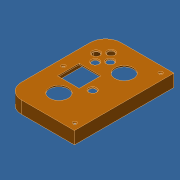
# Autodesk Inventor part: P1704_018_hautManette
Saved by Autodesk Inventor 2019 (Build 230136000, 136)
## iProperties
Created: 2019-05-28
Part Number: P1704_018_hautManette
Project: Nom Projet
Material: .
Description: Nom pièce
Document SubType Name: Modeling
Designer: Adel.KAHRIMANOVIC
Authority: brut Ø
Density: 0.001 g/cm^3
Appearance: Orange
Material number: ---
Author: Adel.KAHRIMANOVIC
Autodesk Inventor part; units mm, degrees
ref_plane "Plan YZ" through (0, 0, 0) normal (1, 0, 0) x (0, 1, 0)
ref_plane "Plan XZ" through (0, 0, 0) normal (0, 1, 0) x (-1, 0, 0)
ref_plane "Plan XY" through (0, 0, 0) normal (0, 0, 1) x (1, 0, 0)
sketch "Esquisse1" plane through (0, 0, 0) normal (0, 0, 1) x (1, 0, 0)
  line L0 (55, 80) -> (55, -80)
  line L1 (-55, -80) -> (-55, 80)
  line L2 (-55, 80) -> (55, -80) construction
  line L3 (55, 80) -> (-55, -80) construction
  line L4 (0, 0) -> (-55, 0) construction
  arc A0 (-55, -55) -> (-30, -80) centre (-30, -55) ccw
  line L5 (-30, -80) -> (55, -80)
  line L6 (-30, -80) -> (-30, -55) construction
  line L7 (55, 80) -> (-30, 80)
  arc A1 (-30, 80) -> (-55, 55) centre (-30, 55) ccw
  line L8 (-30, 55) -> (-30, 80) construction
  line L9 (-83.2132, 0) -> (78.0355, 0) projected
  line L10 (0, -119.2487) -> (0, 119.2487) projected
  dimension "d2" = 160
  dimension "d3" = 110
  dimension "d4" = 25
  dimension "d5" = 25
  constraints: 18 end point, 4 midpoint, 4 point on circle, 3 horizontal, 2 centre point, 2 parallel, 2 point on line, 2 tangent, 2 vertical, 1 collinear, 1 perpendicular
  measures "d2" distance of L0.start L0.end
  measures "d3" distance of L0.end L1.start
  measures "d4" distance of L5.start L6.end
  measures "d5" distance of L8.start L7.end
extrude "Extrusion1" add sketch "Esquisse1" along normal blind 22
sketch "Esquisse6" plane through (0, 0, 0) normal (0, 0, -1) x (-1, 0, 0)
  line L0 (-52.5, 77.5) -> (-52.5, -77.5)
  line L1 (-52.5, -77.5) -> (30, -77.5)
  line L2 (-52.5, 77.5) -> (30, 77.5)
  arc A0 (52.5, 55) -> (30, 77.5) centre (30, 55) ccw
  line L3 (52.5, 55) -> (52.5, -55)
  arc A1 (30, -77.5) -> (52.5, -55) centre (30, -55) ccw
  line L4 (-55, 80) -> (30, 80) projected
  line L5 (-55, -80) -> (-55, 80) projected
  line L6 (30, -80) -> (-55, -80) projected
  line L7 (55, 55) -> (55, -55) projected
  line L8 (30, -239.7653) -> (30, 84.7653) construction
  arc A2 (55, 55) -> (30, 80) centre (30, 55) ccw projected
  line L9 (-55, -80) -> (-55, 80) projected
  line L10 (30, -80) -> (-55, -80) projected
  arc A3 (30, -80) -> (55, -55) centre (30, -55) ccw projected
  line L11 (55, 55) -> (55, -55) projected
  arc A4 (55, 55) -> (30, 80) centre (30, 55) ccw projected
  line L12 (-55, 80) -> (30, 80) projected
  point P0 (0, 0)
  dimension "d8" = 2.5
  dimension "d9" = 2.5
  dimension "d10" = 2.5
  dimension "d11" = 2.5
  constraints: 10 end point, 4 point on circle, 4 tangent, 3 vertical, 2 centre point, 2 point on line, 1 horizontal, 1 midpoint, 1 perpendicular
  measures "d8" distance between parallel lines of L4 L2
  measures "d9" distance between parallel lines of L5 L0
  measures "d10" distance between parallel lines of L6 L1
  measures "d11" distance between parallel lines of L7 L3
extrude "Extrusion2" cut sketch "Esquisse6" against normal blind 2
sketch "Esquisse7" plane through (0, 0, 0) normal (0, 0, -1) x (-1, 0, 0)
  line L0 (-50, 75) -> (-50, -75)
  line L1 (-50, -75) -> (30, -75)
  line L2 (50, 55) -> (50, -55)
  line L3 (-50, 75) -> (30, 75)
  arc A0 (50, 55) -> (30, 75) centre (30, 55) ccw
  arc A1 (30, -75) -> (50, -55) centre (30, -55) ccw
  line L4 (30, 77.5) -> (-52.5, 77.5) projected
  line L5 (-52.5, 77.5) -> (-52.5, -77.5) projected
  line L6 (-52.5, -77.5) -> (30, -77.5) projected
  line L7 (52.5, -55) -> (52.5, 55) projected
  line L8 (30, 77.5) -> (30, 105.4816) construction
  point P0 (0, 0)
  dimension "d14" = 2.5
  dimension "d15" = 2.5
  dimension "d16" = 2.5
  dimension "d17" = 2.5
  constraints: 10 end point, 4 point on circle, 4 tangent, 3 vertical, 2 centre point, 2 point on line, 1 horizontal, 1 perpendicular
  measures "d14" distance between parallel lines of L3 L4
  measures "d15" distance between parallel lines of L5 L0
  measures "d16" distance between parallel lines of L6 L1
  measures "d17" distance between parallel lines of L7 L2
extrude "Extrusion3" cut sketch "Esquisse7" against normal blind 20
sketch "Esquisse8" plane through (0, 0, 22) normal (0, 0, 1) x (1, 0, 0)
  line L0 (-35, -17.5) -> (0, -17.5)
  line L1 (0, -17.5) -> (0, 17.5)
  line L2 (0, 17.5) -> (-35, 17.5)
  line L3 (-35, 17.5) -> (-35, -17.5)
  line L4 (-55, 55) -> (-55, -55) projected
  line L5 (-30, -80) -> (55, -80) projected
  line L6 (-13.2667, 17.5) -> (-13.2667, 80) construction
  line L7 (-17.5, -80) -> (-17.5, -17.5) construction
  line L8 (55, 80) -> (-30, 80) projected
  point P0 (0, 0)
  dimension "d20" = 35
  dimension "d21" = 35
  dimension "d24" = 20
  constraints: 12 end point, 3 parallel, 3 point on line, 2 vertical, 1 horizontal, 1 midpoint, 1 perpendicular
  measures "d20" distance of L2.end L0.start
  measures "d21" distance of L1.end L2.end
  measures "d24" distance between parallel lines of L4 L3
extrude "Extrusion4" cut sketch "Esquisse8" against normal through all
sketch "Esquisse9" plane through (0, 0, 22) normal (0, 0, 1) x (1, 0, 0)
  line L0 (-30, -75) -> (50, -75) projected
  line L1 (-50, 55) -> (-50, -55) projected
  point P0 (0, 0)
  point P1 (44.488, -68.904)
  dimension "d47" = 6.096
  dimension "d48" = 94.488
  measures "d47" distance from line of L0 point (44.488, -68.904)
  measures "d48" distance from line of L1 point (44.488, -68.904)
hole "Perçage1" at (44.488, -68.904, 22) direction (0, 0, -1) diameter 3.4 end through all countersink diameter 6.3 countersink angle 90
sketch "Esquisse10" plane through (0, 0, 22) normal (0, 0, 1) x (1, 0, 0)
  line L0 (-30, -75) -> (50, -75) projected
  line L1 (50, -75) -> (50, 75) projected
  line L2 (-50, 55) -> (-50, -55) projected
  point P0 (0, 0)
  point P1 (43.98, 69.78)
  dimension "d49" = 144.78
  dimension "d51" = 93.98
  measures "d49" distance from line of L0 point (43.98, 69.78)
  measures "d51" distance from line of point (43.98, 69.78) L2
hole "Perçage2" at (43.98, 69.78, 22) direction (0, 0, -1) diameter 3.4 end through all countersink diameter 6.3 countersink angle 90
sketch "Esquisse11" plane through (0, 0, 22) normal (0, 0, 1) x (1, 0, 0)
  line L0 (-30, -75) -> (50, -75) projected
  line L1 (-50, 55) -> (-50, -55) projected
  point P0 (0, 0)
  point P1 (-43.904, 1.2)
  dimension "d52" = 76.2
  dimension "d53" = 6.096
  measures "d52" distance from line of L0 point (-43.904, 1.2)
  measures "d53" distance from line of L1 point (-43.904, 1.2)
hole "Perçage3" at (-43.904, 1.2, 22) direction (0, 0, -1) diameter 3.4 end through all countersink diameter 6.3 countersink angle 90
sketch "Esquisse12" plane through (0, 0, 22) normal (0, 0, 1) x (1, 0, 0)
  circle A0 centre (-10, -40) radius 15
  line L0 (-30, -80) -> (55, -80) projected
  line L1 (-55, 55) -> (-55, -55) projected
  line L2 (-30, -75) -> (50, -75) projected
  line L3 (-50, 55) -> (-50, -55) projected
  circle A1 centre (15, 40) radius 15
  line L4 (50, -75) -> (50, 75) projected
  line L5 (50, 75) -> (-30, 75) projected
  point P0 (0, 0)
  dimension "d58" = 35
  dimension "d59" = 40
  dimension "d60" = 30
  dimension "d61" = 30
  dimension "d62" = 35
  dimension "d63" = 35
  constraints: 2 centre point
  measures "d58" distance from line of L2 A0.centre
  measures "d59" distance from line of A0.centre L3
  measures "d60" diameter of A0
  measures "d61" diameter of A1
  measures "d62" distance from line of L4 A1.centre
  measures "d63" distance from line of L5 A1.centre
extrude "Extrusion6" cut sketch "Esquisse12" against normal through all
sketch "Esquisse13" plane through (0, 0, 22) normal (0, 0, 1) x (1, 0, 0)
  line L0 (-30, -80) -> (55, -80) projected
  line L1 (-55, 55) -> (-55, -55) projected
  point P0 (0, 0)
  point P1 (-35.48, 45.24)
  dimension "d73" = 125.24
  dimension "d74" = 19.52
  measures "d73" distance from line of L0 point (-35.48, 45.24)
  measures "d74" distance from line of L1 point (-35.48, 45.24)
hole "Perçage4" at (-35.48, 45.24, 22) direction (0, 0, -1) diameter 11 end through all countersink diameter 13 countersink angle 90
sketch "Esquisse14" plane through (0, 0, 22) normal (0, 0, 1) x (1, 0, 0)
  line L0 (-30, -80) -> (55, -80) projected
  line L1 (-55, 55) -> (-55, -55) projected
  point P0 (0, 0)
  point P1 (-24.05, 32.535)
  dimension "d96" = 112.535
  dimension "d97" = 30.95
  measures "d96" distance from line of L0 point (-24.05, 32.535)
  measures "d97" distance from line of L1 point (-24.05, 32.535)
hole "Perçage5" at (-24.05, 32.535, 22) direction (0, 0, -1) diameter 11 end through all countersink diameter 13 countersink angle 90
sketch "Esquisse15" plane through (0, 0, 22) normal (0, 0, 1) x (1, 0, 0)
  line L0 (-30, -80) -> (55, -80) projected
  line L1 (-55, 55) -> (-55, -55) projected
  point P0 (0, 0)
  point P1 (-12.62, 45.24)
  dimension "d98" = 125.24
  dimension "d99" = 42.38
  measures "d98" distance from line of L0 point (-12.62, 45.24)
  measures "d99" distance from line of point (-12.62, 45.24) L1
hole "Perçage6" at (-12.62, 45.24, 22) direction (0, 0, -1) diameter 11 end through all countersink diameter 13 countersink angle 90
sketch "Esquisse16" plane through (0, 0, 22) normal (0, 0, 1) x (1, 0, 0)
  line L0 (-55, 55) -> (-55, -55) projected
  line L1 (-30, -80) -> (55, -80) projected
  point P0 (0, 0)
  point P1 (-24.05, 57.935)
  dimension "d100" = 30.95
  dimension "d101" = 137.935
  measures "d100" distance from line of L0 point (-24.05, 57.935)
  measures "d101" distance from line of L1 point (-24.05, 57.935)
hole "Perçage7" at (-24.05, 57.935, 22) direction (0, 0, -1) diameter 11 end through all countersink diameter 13 countersink angle 90
sketch "Esquisse17" plane through (0, 0, 22) normal (0, 0, 1) x (1, 0, 0)
  line L0 (-30, -80) -> (55, -80) projected
  line L1 (55, -80) -> (55, 80) projected
  point P0 (0, 0)
  point P1 (13.128, -8.826)
  dimension "d109" = 71.174
  dimension "d110" = 41.872
  measures "d109" distance from line of L0 point (13.128, -8.826)
  measures "d110" distance from line of L1 point (13.128, -8.826)
hole "Perçage8" at (13.128, -8.826, 22) direction (0, 0, -1) diameter 11 end through all countersink diameter 13 countersink angle 90
